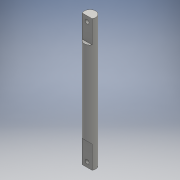
# Autodesk Inventor part: Back axle
Saved by Autodesk Inventor 2016 (Build 200138000, 138)
## iProperties
Created: 2016-02-23
Part Number: Back axle
Material: Generic
Document SubType Name: Modeling
Designer: Michael
Density: 1 g/cm^3
Appearance: Default
Author: Michael
Autodesk Inventor part; units mm, degrees
ref_plane "YZ Plane" through (0, 0, 0) normal (1, 0, 0) x (0, 1, 0)
ref_plane "XZ Plane" through (0, 0, 0) normal (0, 1, 0) x (-1, 0, 0)
ref_plane "XY Plane" through (0, 0, 0) normal (0, 0, 1) x (1, 0, 0)
sketch "Sketch1" plane through (0, 0, 0) normal (0, 0, 1) x (1, 0, 0)
  circle A0 centre (0, 0) radius 3.6
  dimension "d0" = 7.2
  constraints: 1 centre point, 1 coincident
  measures "d0" diameter of A0
extrude "Extrusion1" add sketch "Sketch1" along normal mid plane 83.2
sketch "Sketch2" plane through (0, 0, -41.6) normal (0, 0, -1) x (-1, 0, 0)
  circle A0 centre (0, 0) radius 3.6 projected
  circle A1 centre (0, 0) radius 3.6 projected
  line L0 (3.1168, -1.8015) -> (-3.1186, -1.7985)
  dimension "d3" = 1.8
  constraints: 4 point on circle, 2 end point
  measures "d3" distance from line of point (0, 0) L0
extrude "Extrusion2" cut sketch "Sketch2" against normal blind 14.4 contours L0 A0 picked at (0.0258, -2.6154)
sketch "Sketch3" plane through (3.1186, -1.7985, -41.6) normal (0.0005, -1, 0) x (1, 0.0005, 0)
  line L0 (-3.1177, -16.64) -> (-3.1177, 99.84) projected
  circle A0 centre (-3.1177, 3.2) radius 1.2
  line L1 (0, 0) -> (-6.2354, 0) projected
  point P0 (-3.1177, 41.6)
  dimension "d6" = 2.4
  dimension "d7" = 3.2
  constraints: 1 centre point, 1 point on line
  measures "d6" diameter of A0
  measures "d7" distance from line of L1 A0.centre
extrude "Extrusion3" cut sketch "Sketch3" against normal blind 14.4
mirror "Mirror1" about plane through (0, 0, 0) normal (0, 0, 1) of "Extrusion3", "Extrusion2"
sketch "Sketch4" plane through (0, 0, 0) normal (1, 0, 0) x (0, 1, 0)
  line L0 (-3.6, -27.2) -> (-3.6, 27.2) projected
  line L1 (-1.7985, -27.2) -> (-3.6, -27.2) projected
  line L2 (-1.7985, -27.2) -> (-3.6, -25.3985)
  point P0 (0, 0)
  point P1 (-1.8015, -27.2)
  dimension "d10" = 45
  constraints: 2 end point, 1 point on line
  measures "d10" angle of L1 L2
extrude "Extrusion4" cut sketch "Sketch4" along normal mid plane 14.4
sketch "Sketch5" plane through (0, 0, -41.6) normal (0, 0, -1) x (-1, 0, 0)
  point P0 (0, 0)
sketch "Sketch6" plane through (0, 0, -41.6) normal (0, 0, -1) x (-1, 0, 0)
  line L0 (-3.1186, -1.7985) -> (3.1168, -1.8015) projected
  arc A0 (3.1168, -1.8015) -> (-3.1186, -1.7985) centre (0, 0) ccw projected
  line L1 (-3.1186, -1.7985) -> (3.1168, -1.8015) projected
  arc A1 (3.1168, -1.8015) -> (-3.1186, -1.7985) centre (0, 0) ccw projected
  line L2 (5.2617, -6.8026) -> (-5.2683, -6.7974)
  arc A2 (5.2617, -6.8026) -> (-5.2683, -6.7974) centre (0, 0) ccw
  dimension "d13" = 5
  constraints: 2 end point, 2 point on circle, 1 centre point, 1 other
  measures "d13" distance between parallel lines of L0 L2
extrude "Extrusion5" [suppressed]
body "Solid1"
